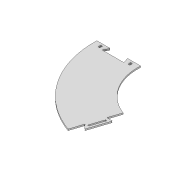
# Autodesk Inventor part: Level 3c - V2
Saved by Autodesk Inventor 2020 (Build 240168000, 168)
## iProperties
Created: 2020-07-30
Part Number: Level 3c - V2
Material: Generic
Document SubType Name: Modeling
Designer: Dan Wikman
Density: 1 g/cm^3
Appearance: Default
Author: Dan Wikman
Autodesk Inventor part; units mm, degrees
ref_plane "YZ Plane" through (0, 0, 0) normal (1, 0, 0) x (0, 1, 0)
ref_plane "XZ Plane" through (0, 0, 0) normal (0, 1, 0) x (-1, 0, 0)
ref_plane "XY Plane" through (0, 0, 0) normal (0, 0, 1) x (1, 0, 0)
sketch "Sketch1" plane through (0, 0, 0) normal (0, 1, 0) x (-1, 0, 0)
  line L0 (0, 0) -> (618.9442, 0)
  line L1 (0, 0) -> (191.2643, 588.6509)
  line L2 (0, 0) -> (-500.7364, 363.8063)
  line L3 (0, 0) -> (-500.7364, -363.8063)
  line L4 (0, 0) -> (191.2643, -588.6509)
  line L5 (396.6438, 3.75) -> (328.1438, 3.75)
  line L6 (328.1438, -3.75) -> (396.6438, -3.75)
  arc A0 (472.3938, 0) -> (145.9777, 449.2732) centre (0, 0) ccw
  arc A1 (77.994, -240.0408) -> (252.3938, 0) centre (0, 0) ccw
  line L7 (289.8938, 3.75) -> (283.8938, 3.75)
  line L8 (283.8938, -3.75) -> (289.8938, -3.75)
  arc A2 (328.1438, 3.75) -> (326.3938, 2) centre (328.1438, 2) ccw
  arc A3 (326.3938, -2) -> (328.1438, -3.75) centre (328.1438, -2) ccw
  line L9 (326.3938, 2) -> (326.3938, -2)
  arc A4 (398.3938, 2) -> (396.6438, 3.75) centre (396.6438, 2) ccw
  arc A5 (396.6438, -3.75) -> (398.3938, -2.0136) centre (396.6573, -2.0136) ccw
  line L10 (398.3938, -2.0136) -> (398.3938, 2)
  line L11 (362.3938, -3.75) -> (362.3938, 32.9806)
  arc A6 (283.8938, 3.75) -> (282.1438, 2) centre (283.8938, 2) ccw
  arc A7 (282.1438, -2) -> (283.8938, -3.75) centre (283.8938, -2) ccw
  arc A8 (289.8938, -3.75) -> (291.6438, -2) centre (289.8938, -2) ccw
  arc A9 (291.6438, 2) -> (289.8938, 3.75) centre (289.8938, 2) ccw
  line L12 (291.6438, 2) -> (291.6438, -2)
  line L13 (282.1438, -2) -> (282.1438, 2)
  line L14 (434.8938, 3.75) -> (440.8938, 3.75)
  line L15 (440.8938, -3.75) -> (434.8938, -3.75)
  arc A10 (442.6438, 2) -> (440.8938, 3.75) centre (440.8938, 2) ccw
  arc A11 (440.8938, -3.75) -> (442.6438, -2) centre (440.8938, -2) ccw
  arc A12 (433.1438, -2) -> (434.8938, -3.75) centre (434.8938, -2) ccw
  arc A13 (434.8938, 3.75) -> (433.1438, 2) centre (434.8938, 2) ccw
  line L16 (433.1438, 2) -> (433.1438, -2)
  line L17 (442.6438, -2) -> (442.6438, 2)
  line L18 (131.9467, 412.5623) -> (135.7509, 411.3262)
  arc A14 (130.8231, 414.7674) -> (131.9467, 412.5623) centre (132.4875, 414.2266) ccw
  arc A15 (135.7509, 411.3262) -> (137.956, 412.4498) centre (136.2917, 412.9905) ccw
  line L19 (139.8101, 418.1561) -> (137.956, 412.4498)
  line L20 (130.8231, 414.7674) -> (132.6772, 420.4737)
  arc A16 (134.8823, 421.5973) -> (132.6772, 420.4737) centre (134.3416, 419.9329) ccw
  line L21 (138.6866, 420.3612) -> (134.8823, 421.5973)
  arc A17 (139.8101, 418.1561) -> (138.6866, 420.3612) centre (138.1458, 418.6969) ccw
  line L22 (125.0255, 378.2728) -> (121.2083, 379.513)
  arc A18 (121.2083, 379.513) -> (119.0032, 378.3895) centre (120.6676, 377.8487) ccw
  arc A19 (126.1361, 376.0718) -> (125.0255, 378.2728) centre (124.4888, 376.6213) ccw
  line L23 (119.0032, 378.3895) -> (97.8355, 313.2421)
  line L24 (98.9591, 311.037) -> (102.7633, 309.8009)
  arc A20 (97.8355, 313.2421) -> (98.9591, 311.037) centre (99.4999, 312.7013) ccw
  arc A21 (102.7633, 309.8009) -> (104.9685, 310.9245) centre (103.3041, 311.4652) ccw
  line L25 (104.9685, 310.9245) -> (126.1361, 376.0718)
  line L26 (88.2208, 277.9878) -> (92.025, 276.7517)
  arc A22 (93.1486, 274.5466) -> (92.025, 276.7517) centre (91.4842, 275.0873) ccw
  line L27 (91.2945, 268.8402) -> (93.1486, 274.5466)
  arc A23 (88.2208, 277.9878) -> (86.0156, 276.8642) centre (87.68, 276.3234) ccw
  line L28 (86.0156, 276.8642) -> (84.1615, 271.1578)
  arc A24 (84.1615, 271.1578) -> (85.2851, 268.9527) centre (85.8259, 270.6171) ccw
  arc A25 (89.0893, 267.7166) -> (91.2945, 268.8402) centre (89.6301, 269.381) ccw
  line L29 (89.0893, 267.7166) -> (85.2851, 268.9527)
  line L30 (-351.5963, 252.9775) -> (-349.2451, 256.2136)
  arc A26 (-354.0407, 252.5903) -> (-351.5963, 252.9775) centre (-353.012, 254.0061) ccw
  arc A27 (-349.2451, 256.2136) -> (-349.6323, 258.658) centre (-350.6609, 257.2422) ccw
  line L31 (-354.4864, 262.1847) -> (-349.6323, 258.658)
  line L32 (-354.0407, 252.5903) -> (-358.8948, 256.1171)
  arc A28 (-359.2819, 258.5615) -> (-358.8948, 256.1171) centre (-357.8661, 257.5328) ccw
  line L33 (-356.9308, 261.7975) -> (-359.2819, 258.5615)
  arc A29 (-354.4864, 262.1847) -> (-356.9308, 261.7975) centre (-355.515, 260.7689) ccw
  line L34 (-321.1238, 235.799) -> (-323.4829, 232.552)
  arc A30 (-323.4829, 232.552) -> (-323.0958, 230.1076) centre (-322.0671, 231.5233) ccw
  arc A31 (-318.6874, 236.1752) -> (-321.1238, 235.799) centre (-319.7189, 234.7783) ccw
  line L35 (-323.0958, 230.1076) -> (-267.6781, 189.8443)
  line L36 (-265.2337, 190.2314) -> (-262.8825, 193.4675)
  arc A32 (-267.6781, 189.8443) -> (-265.2337, 190.2314) centre (-266.6495, 191.26) ccw
  arc A33 (-262.8825, 193.4675) -> (-263.2697, 195.9119) centre (-264.2983, 194.4961) ccw
  line L37 (-263.2697, 195.9119) -> (-318.6874, 236.1752)
  line L38 (-237.1203, 169.8059) -> (-234.7692, 173.0419)
  arc A34 (-232.3248, 173.4291) -> (-234.7692, 173.0419) centre (-233.3534, 172.0133) ccw
  line L39 (-227.4707, 169.9024) -> (-232.3248, 173.4291)
  arc A35 (-237.1203, 169.8059) -> (-236.7332, 167.3615) centre (-235.7046, 168.7773) ccw
  line L40 (-236.7332, 167.3615) -> (-231.8791, 163.8348)
  arc A36 (-231.8791, 163.8348) -> (-229.4347, 164.2219) centre (-230.8505, 165.2505) ccw
  arc A37 (-227.0835, 167.458) -> (-227.4707, 169.9024) centre (-228.4993, 168.4866) ccw
  line L41 (-227.0835, 167.458) -> (-229.4347, 164.2219)
  line L42 (-349.2451, -256.2136) -> (-351.5963, -252.9775)
  arc A38 (-349.6323, -258.658) -> (-349.2451, -256.2136) centre (-350.6609, -257.2422) ccw
  arc A39 (-351.5963, -252.9775) -> (-354.0407, -252.5903) centre (-353.012, -254.0061) ccw
  line L43 (-358.8948, -256.117) -> (-354.0407, -252.5903)
  line L44 (-349.6323, -258.658) -> (-354.4864, -262.1847)
  arc A40 (-356.9308, -261.7975) -> (-354.4864, -262.1847) centre (-355.515, -260.7689) ccw
  line L45 (-359.2819, -258.5615) -> (-356.9308, -261.7975)
  arc A41 (-358.8948, -256.117) -> (-359.2819, -258.5615) centre (-357.8661, -257.5328) ccw
  line L46 (-323.4909, -232.541) -> (-321.1318, -235.788)
  arc A42 (-321.1318, -235.788) -> (-318.6874, -236.1752) centre (-319.716, -234.7594) ccw
  arc A43 (-323.0958, -230.1076) -> (-323.4909, -232.541) centre (-322.086, -231.5203) ccw
  line L47 (-318.6874, -236.1752) -> (-263.2697, -195.9119)
  line L48 (-262.8825, -193.4675) -> (-265.2337, -190.2314)
  arc A44 (-263.2697, -195.9119) -> (-262.8825, -193.4675) centre (-264.2983, -194.4961) ccw
  arc A45 (-265.2337, -190.2314) -> (-267.6781, -189.8443) centre (-266.6495, -191.26) ccw
  line L49 (-267.6781, -189.8443) -> (-323.0958, -230.1076)
  line L50 (-234.7692, -173.0419) -> (-237.1203, -169.8059)
  arc A46 (-236.7332, -167.3615) -> (-237.1203, -169.8059) centre (-235.7046, -168.7773) ccw
  line L51 (-231.8791, -163.8348) -> (-236.7332, -167.3615)
  arc A47 (-234.7692, -173.0419) -> (-232.3248, -173.4291) centre (-233.3534, -172.0133) ccw
  line L52 (-232.3248, -173.4291) -> (-227.4707, -169.9024)
  arc A48 (-227.4707, -169.9024) -> (-227.0835, -167.458) centre (-228.4993, -168.4866) ccw
  arc A49 (-229.4347, -164.2219) -> (-231.8791, -163.8348) centre (-230.8505, -165.2505) ccw
  line L53 (-229.4347, -164.2219) -> (-227.0835, -167.458)
  line L54 (135.7509, -411.3262) -> (131.9467, -412.5623)
  arc A50 (137.956, -412.4498) -> (135.7509, -411.3262) centre (136.2917, -412.9905) ccw
  arc A51 (131.9467, -412.5623) -> (130.8231, -414.7674) centre (132.4875, -414.2266) ccw
  line L55 (132.6772, -420.4737) -> (130.8231, -414.7674)
  line L56 (137.956, -412.4498) -> (139.8101, -418.1561)
  arc A52 (138.6866, -420.3612) -> (139.8101, -418.1561) centre (138.1458, -418.6969) ccw
  line L57 (134.8823, -421.5973) -> (138.6866, -420.3612)
  arc A53 (132.6772, -420.4737) -> (134.8823, -421.5973) centre (134.3416, -419.9329) ccw
  line L58 (121.1954, -379.5172) -> (125.0126, -378.277)
  arc A54 (125.0126, -378.277) -> (126.1361, -376.0718) centre (124.4718, -376.6126) ccw
  arc A55 (119.0032, -378.3895) -> (121.1954, -379.5172) centre (120.6588, -377.8657) ccw
  line L59 (126.1361, -376.0718) -> (104.9685, -310.9245)
  line L60 (102.7633, -309.8009) -> (98.9591, -311.037)
  arc A56 (104.9685, -310.9245) -> (102.7633, -309.8009) centre (103.3041, -311.4652) ccw
  arc A57 (98.9591, -311.037) -> (97.8355, -313.2421) centre (99.4999, -312.7013) ccw
  line L61 (97.8355, -313.2421) -> (119.0032, -378.3895)
  line L62 (92.025, -276.7517) -> (88.2208, -277.9878)
  arc A58 (86.0156, -276.8642) -> (88.2208, -277.9878) centre (87.68, -276.3234) ccw
  line L63 (84.1615, -271.1578) -> (86.0156, -276.8642)
  arc A59 (92.025, -276.7517) -> (93.1486, -274.5466) centre (91.4842, -275.0873) ccw
  line L64 (93.1486, -274.5466) -> (91.2945, -268.8402)
  arc A60 (91.2945, -268.8402) -> (89.0893, -267.7166) centre (89.6301, -269.381) ccw
  arc A61 (85.2851, -268.9527) -> (84.1615, -271.1578) centre (85.8259, -270.6171) ccw
  line L65 (85.2851, -268.9527) -> (89.0893, -267.7166)
  line L66 (-442.5303, 165.2961) -> (-220.837, 122.2033)
  line L67 (-442.5303, -165.2961) -> (-220.837, -122.2033)
  arc A62 (252.3938, 0) -> (-220.837, 122.2033) centre (0, 0) ccw
  arc A63 (-220.837, -122.2033) -> (77.994, -240.0408) centre (0, 0) ccw
  arc A64 (145.9777, 449.2732) -> (-442.5303, 165.2961) centre (0, 0) ccw
  arc A65 (-442.5303, -165.2961) -> (472.3938, 0) centre (0, 0) ccw
  line L68 (115.6782, 400.5167) -> (82.9862, 299.9012)
  line L69 (84.6505, 297.6104) -> (108.7484, 297.6104)
  line L70 (110.4128, 295.3196) -> (90.9552, 235.4353)
  line L71 (138.8662, 382.8904) -> (158.9929, 444.8338)
  line L72 (118.6344, 401.1564) -> (135.91, 382.2507)
  line L73 (123.1169, 378.8929) -> (127.2722, 391.7035) construction
  line L74 (100.8612, 310.4189) -> (96.6995, 297.6104) construction
  arc A66 (135.91, 382.2507) -> (138.8662, 382.8904) centre (137.2019, 383.4311) ccw
  arc A67 (118.6344, 401.1564) -> (115.6782, 400.5167) centre (117.3425, 399.9759) ccw
  arc A68 (82.9862, 299.9012) -> (84.6505, 297.6104) centre (84.6505, 299.3604) ccw
  arc A69 (110.4128, 295.3196) -> (108.7484, 297.6104) centre (108.7484, 295.8604) ccw
  line L75 (407.0624, -13.75) -> (472.1936, -13.75)
  arc A70 (405.5405, -11.1361) -> (407.0624, -13.75) centre (407.0624, -12) ccw
  line L76 (418.1824, 11.1361) -> (405.5405, -11.1361)
  arc A71 (418.1824, 11.1361) -> (416.6605, 13.75) centre (416.6605, 12) ccw
  line L77 (416.6605, 13.75) -> (310.8671, 13.75)
  line L78 (309.2028, 11.4592) -> (316.6494, -11.4592)
  arc A72 (310.8671, 13.75) -> (309.2028, 11.4592) centre (310.8671, 12) ccw
  arc A73 (314.9851, -13.75) -> (316.6494, -11.4592) centre (314.9851, -12) ccw
  line L79 (314.9851, -13.75) -> (252.019, -13.75)
  line L80 (112.7122, -391.3883) -> (132.8388, -453.3318)
  arc A74 (114.7278, -389.1332) -> (112.7122, -391.3883) centre (114.3765, -390.8476) ccw
  line L81 (139.8166, -394.2739) -> (114.7278, -389.1332)
  arc A75 (139.8166, -394.2739) -> (141.8322, -392.0187) centre (140.1679, -392.5595) ccw
  line L82 (141.8322, -392.0187) -> (109.1403, -291.4032)
  line L83 (106.4473, -290.5282) -> (86.9517, -304.6926)
  arc A76 (109.1403, -291.4032) -> (106.4473, -290.5282) centre (107.4759, -291.944) ccw
  arc A77 (84.2587, -303.8176) -> (86.9517, -304.6926) centre (85.9231, -303.2768) ccw
  line L84 (84.2587, -303.8176) -> (64.8011, -243.9333)
  line L85 (-359.2819, 258.5615) -> (-362.9556, 253.5051)
  line L86 (-362.5684, 251.0607) -> (-357.7143, 247.534)
  line L87 (-351.5963, 252.9775) -> (-355.2699, 247.9211)
  arc A78 (-362.9556, 253.5051) -> (-362.5684, 251.0607) centre (-361.5398, 252.4765) ccw
  arc A79 (-357.7143, 247.534) -> (-355.2699, 247.9211) centre (-356.6857, 248.9498) ccw
  line L88 (-237.1203, 169.8059) -> (-240.794, 164.7495)
  line L89 (-240.4068, 162.3051) -> (-235.5527, 158.7784)
  line L90 (-229.4347, 164.2219) -> (-233.1083, 159.1656)
  arc A80 (-240.794, 164.7495) -> (-240.4068, 162.3051) centre (-239.3782, 163.7209) ccw
  arc A81 (-235.5527, 158.7784) -> (-233.1083, 159.1656) centre (-234.5241, 160.1942) ccw
  line L91 (-356.9308, -261.7975) -> (-353.2571, -266.8539)
  arc A82 (-353.2571, -266.8539) -> (-350.8127, -267.241) centre (-351.8413, -265.8253) ccw
  line L92 (-350.8127, -267.241) -> (-345.9586, -263.7143)
  arc A83 (-345.9586, -263.7143) -> (-345.5715, -261.2699) centre (-346.9872, -262.2985) ccw
  line L93 (-349.2451, -256.2136) -> (-345.5715, -261.2699)
  line L94 (-234.7692, -173.0419) -> (-231.0955, -178.0983)
  arc A84 (-231.0955, -178.0983) -> (-228.6511, -178.4855) centre (-229.6798, -177.0697) ccw
  line L95 (-228.6511, -178.4855) -> (-223.797, -174.9587)
  arc A85 (-223.797, -174.9587) -> (-223.4099, -172.5143) centre (-224.8257, -173.543) ccw
  line L96 (-227.0835, -167.458) -> (-223.4099, -172.5143)
  line L97 (138.6866, -420.3612) -> (144.6307, -418.4299)
  arc A86 (144.6307, -418.4299) -> (145.7542, -416.2247) centre (144.0899, -416.7655) ccw
  line L98 (145.7542, -416.2247) -> (143.9001, -410.5184)
  arc A87 (143.9001, -410.5184) -> (141.695, -409.3948) centre (142.2358, -411.0592) ccw
  line L99 (135.7509, -411.3262) -> (141.695, -409.3948)
  line L100 (92.025, -276.7517) -> (97.9691, -274.8203)
  arc A88 (97.9691, -274.8203) -> (99.0927, -272.6152) centre (97.4283, -273.156) ccw
  line L101 (99.0927, -272.6152) -> (97.2386, -266.9089)
  arc A89 (97.2386, -266.9089) -> (95.0334, -265.7853) centre (95.5742, -267.4496) ccw
  line L102 (89.0893, -267.7166) -> (95.0334, -265.7853)
  line L103 (442.6438, 2) -> (442.6438, 8.25)
  arc A90 (442.6438, 8.25) -> (440.8938, 10) centre (440.8938, 8.25) ccw
  line L104 (440.8938, 10) -> (434.8938, 10)
  arc A91 (434.8938, 10) -> (433.1438, 8.25) centre (434.8938, 8.25) ccw
  line L105 (433.1438, 2) -> (433.1438, 8.25)
  line L106 (291.6438, 2) -> (291.6438, 8.25)
  arc A92 (291.6438, 8.25) -> (289.8938, 10) centre (289.8938, 8.25) ccw
  line L107 (289.8938, 10) -> (283.8938, 10)
  arc A93 (283.8938, 10) -> (282.1438, 8.25) centre (283.8938, 8.25) ccw
  line L108 (282.1438, 2) -> (282.1438, 8.25)
  line L109 (134.8823, 421.5973) -> (128.9382, 423.5286)
  arc A94 (128.9382, 423.5286) -> (126.7331, 422.4051) centre (128.3975, 421.8643) ccw
  line L110 (126.7331, 422.4051) -> (124.879, 416.6987)
  arc A95 (124.879, 416.6987) -> (126.0026, 414.4936) centre (126.5434, 416.158) ccw
  line L111 (131.9467, 412.5623) -> (126.0026, 414.4936)
  line L112 (88.2208, 277.9878) -> (82.2767, 279.9191)
  arc A96 (82.2767, 279.9191) -> (80.0715, 278.7955) centre (81.7359, 278.2548) ccw
  line L113 (80.0715, 278.7955) -> (78.2174, 273.0892)
  arc A97 (78.2174, 273.0892) -> (79.341, 270.8841) centre (79.8818, 272.5484) ccw
  line L114 (85.2851, 268.9527) -> (79.341, 270.8841)
  point P0 (115.5523, 343.4982)
  point P1 (-290.9785, 216.0435)
  point P2 (-295.3869, -209.9759)
  point P3 (108.4194, -345.8158)
  point P4 (137.9375, 380.0319)
  point P5 (97.9406, 311.9068)
  point P6 (104.0986, 309.906)
  point P7 (119.8731, 379.408)
  point P8 (404.0568, -13.75)
  point P9 (411.8615, 0)
  point P10 (312.9261, 0)
  point P11 (111.7834, -388.5299)
  point P12 (127.2722, -391.7035)
  point P13 (96.6995, -297.6104)
  point P14 (282.1438, 2)
  point P15 (442.6438, 2)
  dimension "d4" = 360
  dimension "d6" = 7.5
  dimension "d7" = 7.5
  dimension "d9" = 68.5
  dimension "d10" = 7.5
  dimension "d11" = 7.5
  dimension "d12" = 3.5
  dimension "d13" = 3.5
  dimension "d19" = 360
  dimension "d21" = 25
  dimension "d25" = 10
  dimension "d26" = 10
  dimension "d27" = 1.75
  dimension "d30" = 144
  dimension "d34" = 0
  dimension "d35" = 8
  dimension "d36" = 1.75
  dimension "d43" = 8
  dimension "d44" = 1.75
  dimension "d47" = 360
  constraints: 230 end point, 201 point on circle, 98 centre point, 23 tangent, 16 point on line, 14 symmetric about line, 5 equal radius, 5 midpoint, 4 horizontal, 4 parallel, 2 coincident, 2 vertical, 1 collinear, 1 equal length, 517 other
  measures "d6" distance between parallel lines of L5 L6
  measures "d7" diameter of L6 L0
  measures "d9" distance of L6.start L6.end
  measures "d10" distance between parallel lines of L7 L8
  measures "d11" diameter of L7 L0
  measures "d12" diameter of A2
  measures "d13" diameter of A3
  measures "d21" angle of L35 L66
  measures "d25" distance between parallel lines of L23 L68
  measures "d26" distance between parallel lines of L25 L70
  measures "d27" radius of A66
  measures "d34" angle of L32 L86
  measures "d35" distance from line of L33.end L86
  measures "d36" radius of A78
  measures "d43" distance from line of L88.start L89
  measures "d44" radius of A80
extrude "Extrusion1" add sketch "Sketch1" along normal blind 7 contours A62 L70 A69 L69 L1 L24 A21 L25 A19 L22 L72 A66 L71 A0 L0 L17 L103 A90 L104 A91 L105 L16 L76 A71 L77 A72 L78 L12 L106 A92 L107 A93 L108 L13 | L0 L13 A7 L8 A8 L12 L78 A73 L79 A1 | L69 A68 L68 A67 L72 L1 L22 A18 L23 A20 L24 | A65 L75 A70 L76 L0 L16 A12 L15 A11 L17
body "Solid1"
